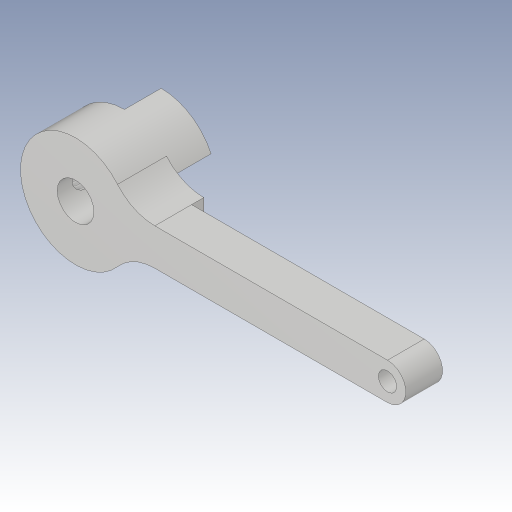
# Autodesk Inventor part: BT006_huenin20_23
Saved by Autodesk Inventor 2023.3 (Build 273359000, 359)
## iProperties
Company: HTBLA Kaindorf
RuleStatus: InUse
Created: 2024-04-11
Part Number: BT006_huenin20_23
Project: Fiberprinter-Hotend
Material: Aluminium
Description: Schneidhebel
Document SubType Name: Modeling
Designer: huenin20
Density: 2.7 g/cm^3
Appearance: Satin
Mass: 1.31798 g
Surface Area: 6.32402 cm^2
Volume: 0.48814 cm^3
AfterDocNew0: iProperties-Editor_aufrufen
Author: nicob
Keywords: 2023
Autodesk Inventor part; units mm, degrees
ref_plane "YZ Plane" through (0, 0, 0) normal (1, 0, 0) x (0, 1, 0)
ref_plane "XY Plane" through (0, 0, 0) normal (0, 0, 1) x (1, 0, 0)
sketch "Skizze3" plane through (0, 0, 0) normal (1, 0, 0) x (0, 1, 0)
  circle A0 centre (0, 0) radius 1.5
  circle A1 centre (0, 0) radius 4.5
  line L0 (4.2426, 1.5) -> (27, 1.5)
  line L1 (27, 1.5) -> (27, -1.5)
  line L2 (27, -1.5) -> (4.2426, -1.5)
  point P0 (27, 0)
  point P1 (0, 4.5)
  point P2 (25.5, 0)
  dimension "d4" = 3
  dimension "d5" = 9
  dimension "d6" = 3
  dimension "d7" = 27
  dimension "d25" = 1.5
  constraints: 6 end point, 3 point on circle, 2 centre point, 2 coincident, 2 horizontal alignment, 2 perpendicular, 1 horizontal, 1 midpoint, 1 vertical alignment
  measures "d4" diameter of A0
  measures "d5" diameter of A1
  measures "d6" distance of L0.end L1.end
  measures "d7" distance from line of L1 point (0, 0)
  measures "d25" distance from line of L1 point (25.5, 0)
extrude "Extrusion3" add sketch "Skizze3" along normal blind 4
fillet "Rundung1" radius 4 2 edges at (2, 4.2426, 1.5) (2, 4.2426, -1.5)
ref_plane "Arbeitsebene1" through (0, -4.5, 0) normal (0, 1, 0) x (-1, 0, 0)
sketch "Skizze4" plane through (0, -4.5, 0) normal (0, 1, 0) x (-1, 0, 0)
  line L0 (0, 4.5) -> (-4, 4.5) projected
  point P0 (0, 0)
  point P1 (-2, 0)
  point P2 (-2, 4.5)
  constraints: 1 horizontal alignment, 1 midpoint, 1 vertical alignment
hole "Bohrung1" at (2, -4.5, 0) direction (0, 1, 0) diameter 1.567 depth 4.5 thread size "M2x0.4" class "6H" standard "ISO Metric profile"
sketch "Skizze5" plane through (0, 0, 0) normal (-1, 0, 0) x (0, 0, 1)
  line L0 (1.5, 27) -> (1.5, 6.4807) projected
  line L1 (-1.5, 27) -> (1.5, 27) projected
  line L2 (-1.5, 6.4807) -> (-1.5, 27) projected
  arc A0 (-2.9118, 3.431) -> (-1.5, 6.4807) centre (-5.5, 6.4807) ccw projected
  arc A1 (-2.9118, 3.431) -> (2.9118, 3.431) centre (0, 0) ccw projected
  arc A2 (1.5, 6.4807) -> (2.9118, 3.431) centre (5.5, 6.4807) ccw projected
  circle A3 centre (0, 0) radius 1.5 projected
  line L3 (4.5, 0) -> (-4.5, 0)
  line L4 (-1.9018, -4.0784) -> (1.9018, 4.0784)
  line L5 (0, 0) -> (0, 4.5) construction
  circle A4 centre (0, 0) radius 4.5
  point P0 (0.6339, 1.3595)
  point P1 (1.5, 0)
  point P2 (-0.6339, -1.3595)
  point P3 (-1.5, 0)
  dimension "d24" = 25
  constraints: 6 end point, 6 point on circle, 3 midpoint, 1 centre point, 1 coincident, 1 horizontal, 1 perpendicular
  measures "d24" angle of L5 L4
extrude "Extrusion4" add sketch "Skizze5" along normal blind 3 contours A1 L3 A3 L4 A4 | A1 L3 A3 L4 picked at (3.4649, 0.3226) picked at (-2.9025, -1.9162)
hole "Bohrung2" at (0, 25.5, 0) direction (1, 0, 0) diameter 1.5 end through all
fillet "Rundung2" radius 1.5 2 edges at (2, 27, 1.5) (2, 27, -1.5)
sketch "Skizze6" plane through (0, 0, 0) normal (-1, 0, 0) x (0, 0, 1)
  arc A0 (1.5, 25.5) -> (-1.5, 25.5) centre (0, 25.5) ccw projected
  line L0 (-1.5, 6.4807) -> (-1.5, 25.5) projected
  arc A1 (-2.9118, 3.431) -> (-1.5, 6.4807) centre (-5.5, 6.4807) ccw projected
  arc A2 (-2.9118, 3.431) -> (-4.5, 0) centre (0, 0) ccw projected
  line L1 (-4.5, 0) -> (-1.5, 0) projected
  arc A3 (0.6339, 1.3595) -> (-1.5, 0) centre (0, 0) ccw projected
  line L2 (0.6339, 1.3595) -> (1.9018, 4.0784) projected
  arc A4 (2.9118, 3.431) -> (1.9018, 4.0784) centre (0, 0) ccw projected
  arc A5 (1.5, 6.4807) -> (2.9118, 3.431) centre (5.5, 6.4807) ccw projected
  line L3 (1.5, 25.5) -> (1.5, 6.4807) projected
  circle A6 centre (0, 25.5) radius 0.75 projected
  line L4 (1.5, 25.5) -> (1.5, 6.4807) projected
  line L5 (1.5, 15.9904) -> (-1.5, 15.9904)
  line L6 (-1.5, 6.4807) -> (-1.5, 25.5) projected
  line L7 (1.5, 25.5) -> (1.5, 6.4807) projected
  line L8 (1.5, 6.4807) -> (-1.5, 6.4807)
  constraints: 4 end point, 2 midpoint, 1 perpendicular
extrude "Extrusion5" cut sketch "Skizze6" against normal blind 1 contours L3 L5 L0 A0 | L3 L8 L0 L5
equation "\"d25\" = 0.5 * d6"
equation "\"d12\" = 0.5 * d5"
equation "\"d16\" = 0.5 * d5"
equation "\"d27\" = 0.5 * d5"
equation "\"d31\" = 0.5 * d5"
